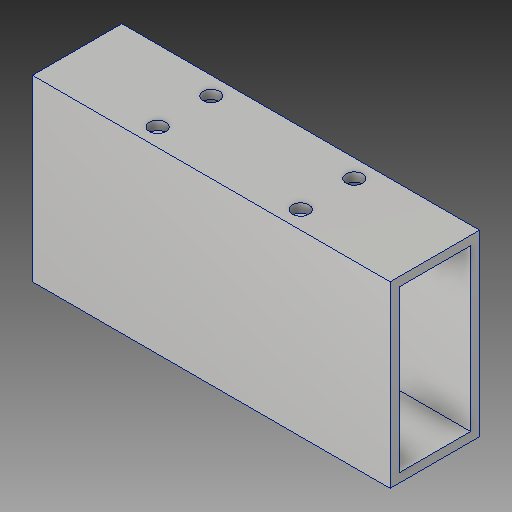
# Autodesk Inventor part: SmallSupportExtrusion
Saved by Autodesk Inventor 2019.4 (Build 234330000, 330)
## iProperties
Created: 2020-01-02
Part Number: SmallSupportExtrusion
Material: Aluminum 6061
Document SubType Name: Modeling
Designer: Mark
Mass: 161.756 g
Surface Area: 413.626 cm^2
Volume: 59.9098 cm^3
Density: 2.7 g/cm^3
Appearance: Aluminum - Flat
Author: Mark
Autodesk Inventor part; units mm, degrees
ref_plane "YZ Plane" through (0, 0, 0) normal (1, 0, 0) x (0, 1, 0)
ref_plane "XZ Plane" through (0, 0, 0) normal (0, 1, 0) x (-1, 0, 0)
ref_plane "XY Plane" through (0, 0, 0) normal (0, 0, 1) x (1, 0, 0)
sketch "Sketch1" plane through (0, 0, 0) normal (1, 0, 0) x (0, 1, 0)
  line L0 (-30, 15) -> (30, 15)
  line L1 (30, 15) -> (30, -15)
  line L2 (30, -15) -> (-30, -15)
  line L3 (-30, -15) -> (-30, 15)
  line L4 (-30, 15) -> (30, -15) construction
  line L5 (30, 15) -> (-30, -15) construction
  line L6 (-27, 12) -> (27, 12)
  line L7 (27, 12) -> (27, -12)
  line L8 (27, -12) -> (-27, -12)
  line L9 (-27, -12) -> (-27, 12)
  line L10 (-27, 12) -> (27, -12) construction
  line L11 (27, 12) -> (-27, -12) construction
  point P0 (0, 0)
  dimension "d0" = 60
  dimension "d1" = 30
  dimension "d2" = 54
  dimension "d3" = 24
  constraints: 24 end point, 4 midpoint, 4 parallel, 2 horizontal, 2 perpendicular
  measures "d0" distance of L1.end L2.end
  measures "d1" distance of L0.end L1.end
  measures "d2" distance of L7.end L8.end
  measures "d3" distance of L6.end L7.end
extrude "Extrusion1" add sketch "Sketch1" along normal blind 120
sketch "Sketch2" plane through (0, 30, 15) normal (0, 1, 0) x (1, 0, 0)
  circle A0 centre (36, 6) radius 2.75
  circle A1 centre (36, 24) radius 2.75
  circle A2 centre (84, 6) radius 2.75
  circle A3 centre (84, 24) radius 2.75
  line L0 (0, 30) -> (120, 30) projected
  line L1 (0, 0) -> (0, 30) projected
  point P0 (0, 15)
  dimension "d6" = 5.5
  dimension "d7" = 5.5
  dimension "d8" = 5.5
  dimension "d9" = 5.5
  dimension "d10" = 18
  dimension "d11" = 48
  dimension "d12" = 18
  dimension "d13" = 48
  dimension "d14" = 6
  dimension "d15" = 6
  dimension "d16" = 48
  dimension "d17" = 36
  constraints: 4 centre point
  measures "d6" diameter of A0
  measures "d7" diameter of A1
  measures "d8" diameter of A2
  measures "d9" diameter of A3
  measures "d10" distance of A2.centre A3.centre
  measures "d11" distance of A1.centre A3.centre
  measures "d12" distance of A0.centre A1.centre
  measures "d13" distance of A2.centre A0.centre
  measures "d14" distance from line of L0 A1.centre
  measures "d15" distance from line of L0 A3.centre
  measures "d16" horizontal distance of A3.centre A0.centre
  measures "d17" distance from line of L1 A0.centre
extrude "Extrusion2" cut sketch "Sketch2" against normal up to surface (60 mm away)
body "Solid1"
